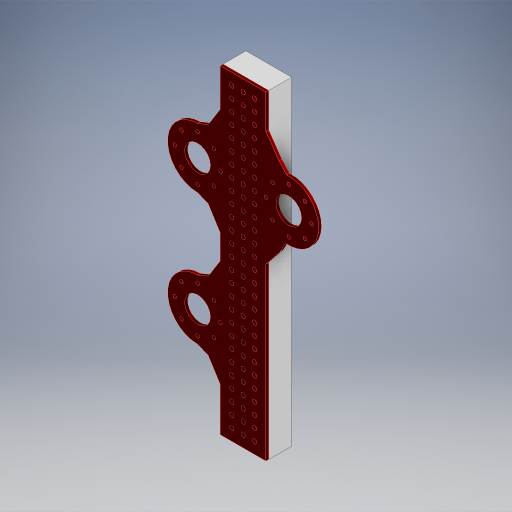
# Autodesk Inventor part: 2024-210-008-Shooter-Gusset-Plate
Saved by Autodesk Inventor 2024.2 (Build 282272000, 272)
## iProperties
Created: 2024-02-16
Part Number: 2024-210-008-Shooter-Gusset-Plate
Material: Generic
Document SubType Name: Modeling
Designer: rohan
Density: 1 g/cm^3
Appearance: Default
Author: rohan
Autodesk Inventor part; units mm, degrees
ref_plane "YZ Plane" through (0, 0, 0) normal (1, 0, 0) x (0, 1, 0)
ref_plane "XZ Plane" through (0, 0, 0) normal (0, 1, 0) x (-1, 0, 0)
ref_plane "XY Plane" through (0, 0, 0) normal (0, 0, 1) x (1, 0, 0)
sketch "Sketch1" plane through (0, 0, 0) normal (0, 1, 0) x (-1, 0, 0)
  line L0 (25.4, 12.7) -> (-25.4, 12.7)
  line L1 (-25.4, 12.7) -> (-25.4, -12.7)
  line L2 (-25.4, -12.7) -> (25.4, -12.7)
  line L3 (25.4, -12.7) -> (25.4, 12.7)
  line L4 (25.4, 12.7) -> (-25.4, -12.7) construction
  line L5 (-25.4, 12.7) -> (25.4, -12.7) construction
  point P0 (0, 0)
  dimension "d0" = 50.8
  dimension "d1" = 25.4
  constraints: 12 end point, 2 midpoint, 2 parallel, 1 horizontal, 1 perpendicular
  measures "d0" distance of L2.end L1.end
  measures "d1" distance of L1.end L0.end
extrude "Extrusion1" add sketch "Sketch1" along normal blind 355.6
sketch "Sketch2" plane through (-25.4, 0, 12.7) normal (0, 0, 1) x (1, 0, 0)
  circle A0 centre (12.7, 12.7) radius 2.4892
  line L0 (0, 0) -> (0, 355.6) projected
  line L1 (0, 0) -> (50.8, 0) projected
  circle A1 centre (25.4, 12.7) radius 2.4892
  circle A2 centre (38.1, 12.7) radius 2.4892
  circle A3 centre (12.7, 25.4) radius 2.4892
  circle A4 centre (25.4, 25.4) radius 2.4892
  circle A5 centre (38.1, 25.4) radius 2.4892
  circle A6 centre (12.7, 38.1) radius 2.4892
  circle A7 centre (25.4, 38.1) radius 2.4892
  circle A8 centre (38.1, 38.1) radius 2.4892
  circle A9 centre (12.7, 50.8) radius 2.4892
  circle A10 centre (25.4, 50.8) radius 2.4892
  circle A11 centre (38.1, 50.8) radius 2.4892
  circle A12 centre (12.7, 63.5) radius 2.4892
  circle A13 centre (25.4, 63.5) radius 2.4892
  circle A14 centre (38.1, 63.5) radius 2.4892
  circle A15 centre (12.7, 76.2) radius 2.4892
  circle A16 centre (25.4, 76.2) radius 2.4892
  circle A17 centre (38.1, 76.2) radius 2.4892
  circle A18 centre (12.7, 88.9) radius 2.4892
  circle A19 centre (25.4, 88.9) radius 2.4892
  circle A20 centre (38.1, 88.9) radius 2.4892
  circle A21 centre (12.7, 101.6) radius 2.4892
  circle A22 centre (25.4, 101.6) radius 2.4892
  circle A23 centre (38.1, 101.6) radius 2.4892
  circle A24 centre (12.7, 114.3) radius 2.4892
  circle A25 centre (25.4, 114.3) radius 2.4892
  circle A26 centre (38.1, 114.3) radius 2.4892
  circle A27 centre (12.7, 127) radius 2.4892
  circle A28 centre (25.4, 127) radius 2.4892
  circle A29 centre (38.1, 127) radius 2.4892
  circle A30 centre (12.7, 139.7) radius 2.4892
  circle A31 centre (25.4, 139.7) radius 2.4892
  circle A32 centre (38.1, 139.7) radius 2.4892
  circle A33 centre (12.7, 152.4) radius 2.4892
  circle A34 centre (25.4, 152.4) radius 2.4892
  circle A35 centre (38.1, 152.4) radius 2.4892
  circle A36 centre (12.7, 165.1) radius 2.4892
  circle A37 centre (25.4, 165.1) radius 2.4892
  circle A38 centre (38.1, 165.1) radius 2.4892
  circle A39 centre (12.7, 177.8) radius 2.4892
  circle A40 centre (25.4, 177.8) radius 2.4892
  circle A41 centre (38.1, 177.8) radius 2.4892
  circle A42 centre (12.7, 190.5) radius 2.4892
  circle A43 centre (25.4, 190.5) radius 2.4892
  circle A44 centre (38.1, 190.5) radius 2.4892
  circle A45 centre (12.7, 203.2) radius 2.4892
  circle A46 centre (25.4, 203.2) radius 2.4892
  circle A47 centre (38.1, 203.2) radius 2.4892
  circle A48 centre (12.7, 215.9) radius 2.4892
  circle A49 centre (25.4, 215.9) radius 2.4892
  circle A50 centre (38.1, 215.9) radius 2.4892
  circle A51 centre (12.7, 228.6) radius 2.4892
  circle A52 centre (25.4, 228.6) radius 2.4892
  circle A53 centre (38.1, 228.6) radius 2.4892
  circle A54 centre (12.7, 241.3) radius 2.4892
  circle A55 centre (25.4, 241.3) radius 2.4892
  circle A56 centre (38.1, 241.3) radius 2.4892
  circle A57 centre (12.7, 254) radius 2.4892
  circle A58 centre (25.4, 254) radius 2.4892
  circle A59 centre (38.1, 254) radius 2.4892
  circle A60 centre (12.7, 266.7) radius 2.4892
  circle A61 centre (25.4, 266.7) radius 2.4892
  circle A62 centre (38.1, 266.7) radius 2.4892
  circle A63 centre (12.7, 279.4) radius 2.4892
  circle A64 centre (25.4, 279.4) radius 2.4892
  circle A65 centre (38.1, 279.4) radius 2.4892
  circle A66 centre (12.7, 292.1) radius 2.4892
  circle A67 centre (25.4, 292.1) radius 2.4892
  circle A68 centre (38.1, 292.1) radius 2.4892
  circle A69 centre (12.7, 304.8) radius 2.4892
  circle A70 centre (25.4, 304.8) radius 2.4892
  circle A71 centre (38.1, 304.8) radius 2.4892
  circle A72 centre (12.7, 317.5) radius 2.4892
  circle A73 centre (25.4, 317.5) radius 2.4892
  circle A74 centre (38.1, 317.5) radius 2.4892
  circle A75 centre (12.7, 330.2) radius 2.4892
  circle A76 centre (25.4, 330.2) radius 2.4892
  circle A77 centre (38.1, 330.2) radius 2.4892
  circle A78 centre (12.7, 342.9) radius 2.4892
  circle A79 centre (25.4, 342.9) radius 2.4892
  circle A80 centre (38.1, 342.9) radius 2.4892
  point P0 (25.4, 0)
  dimension "d4" = 4.9784
  dimension "d5" = 12.7
  dimension "d6" = 12.7
  dimension "d9" = 12.7
  dimension "d12" = 12.7
  constraints: 81 centre point, 1 horizontal, 1 vertical, 160 other
  measures "d4" diameter of A0
  measures "d5" distance from line of A0.centre L1
  measures "d6" distance from line of L0 A0.centre
  measures "d9" distance of A0.centre A1.centre
  measures "d12" distance of A0.centre A3.centre
extrude "Extrusion2" cut sketch "Sketch2" against normal blind 355.6
sketch "Sketch3" plane through (-25.4, 0, 12.7) normal (0, 0, 1) x (1, 0, 0)
  circle A0 centre (38.1, 342.9) radius 2.4892 projected
  circle A1 centre (12.7, 317.5) radius 2.4892 projected
  circle A2 centre (12.7, 292.1) radius 2.4892 projected
  circle A3 centre (38.1, 266.7) radius 2.4892 projected
  circle A4 centre (25.4, 304.8) radius 2.4892 projected
  circle A5 centre (12.7, 241.3) radius 2.4892 projected
  circle A6 centre (38.1, 215.9) radius 2.4892 projected
  circle A7 centre (38.1, 254) radius 2.4892 projected
  circle A8 centre (25.4, 203.2) radius 2.4892 projected
  circle A9 centre (38.1, 177.8) radius 2.4892 projected
  circle A10 centre (38.1, 165.1) radius 2.4892 projected
  circle A11 centre (12.7, 165.1) radius 2.4892 projected
  circle A12 centre (25.4, 127) radius 2.4892 projected
  circle A13 centre (38.1, 114.3) radius 2.4892 projected
  circle A14 centre (12.7, 88.9) radius 2.4892 projected
  circle A15 centre (25.4, 101.6) radius 2.4892 projected
  circle A16 centre (38.1, 63.5) radius 2.4892 projected
  circle A17 centre (12.7, 50.8) radius 2.4892 projected
  circle A18 centre (38.1, 12.7) radius 2.4892 projected
  circle A19 centre (12.7, 38.1) radius 2.4892 projected
  circle A20 centre (25.4, 38.1) radius 2.4892 projected
  circle A21 centre (25.4, 12.7) radius 2.4892 projected
  circle A22 centre (12.7, 63.5) radius 2.4892 projected
  circle A23 centre (38.1, 50.8) radius 2.4892 projected
  circle A24 centre (38.1, 101.6) radius 2.4892 projected
  circle A25 centre (12.7, 76.2) radius 2.4892 projected
  circle A26 centre (25.4, 114.3) radius 2.4892 projected
  circle A27 centre (25.4, 139.7) radius 2.4892 projected
  circle A28 centre (12.7, 152.4) radius 2.4892 projected
  circle A29 centre (38.1, 152.4) radius 2.4892 projected
  circle A30 centre (25.4, 177.8) radius 2.4892 projected
  circle A31 centre (38.1, 203.2) radius 2.4892 projected
  circle A32 centre (25.4, 254) radius 2.4892 projected
  circle A33 centre (38.1, 228.6) radius 2.4892 projected
  circle A34 centre (12.7, 228.6) radius 2.4892 projected
  circle A35 centre (38.1, 292.1) radius 2.4892 projected
  circle A36 centre (25.4, 279.4) radius 2.4892 projected
  circle A37 centre (12.7, 279.4) radius 2.4892 projected
  circle A38 centre (25.4, 317.5) radius 2.4892 projected
  circle A39 centre (12.7, 330.2) radius 2.4892 projected
  circle A40 centre (25.4, 342.9) radius 2.4892 projected
  circle A41 centre (38.1, 330.2) radius 2.4892 projected
  circle A42 centre (12.7, 304.8) radius 2.4892 projected
  circle A43 centre (25.4, 266.7) radius 2.4892 projected
  circle A44 centre (25.4, 292.1) radius 2.4892 projected
  circle A45 centre (12.7, 254) radius 2.4892 projected
  circle A46 centre (25.4, 215.9) radius 2.4892 projected
  circle A47 centre (38.1, 241.3) radius 2.4892 projected
  circle A48 centre (12.7, 203.2) radius 2.4892 projected
  circle A49 centre (25.4, 190.5) radius 2.4892 projected
  circle A50 centre (38.1, 190.5) radius 2.4892 projected
  circle A51 centre (25.4, 152.4) radius 2.4892 projected
  circle A52 centre (12.7, 127) radius 2.4892 projected
  circle A53 centre (38.1, 127) radius 2.4892 projected
  circle A54 centre (12.7, 101.6) radius 2.4892 projected
  circle A55 centre (25.4, 88.9) radius 2.4892 projected
  circle A56 centre (38.1, 76.2) radius 2.4892 projected
  circle A57 centre (25.4, 63.5) radius 2.4892 projected
  circle A58 centre (38.1, 25.4) radius 2.4892 projected
  circle A59 centre (12.7, 25.4) radius 2.4892 projected
  circle A60 centre (25.4, 25.4) radius 2.4892 projected
  circle A61 centre (12.7, 12.7) radius 2.4892 projected
  circle A62 centre (38.1, 38.1) radius 2.4892 projected
  circle A63 centre (25.4, 50.8) radius 2.4892 projected
  circle A64 centre (38.1, 88.9) radius 2.4892 projected
  circle A65 centre (25.4, 76.2) radius 2.4892 projected
  circle A66 centre (12.7, 114.3) radius 2.4892 projected
  circle A67 centre (38.1, 139.7) radius 2.4892 projected
  circle A68 centre (12.7, 139.7) radius 2.4892 projected
  circle A69 centre (25.4, 165.1) radius 2.4892 projected
  circle A70 centre (12.7, 177.8) radius 2.4892 projected
  circle A71 centre (12.7, 190.5) radius 2.4892 projected
  circle A72 centre (25.4, 228.6) radius 2.4892 projected
  circle A73 centre (25.4, 241.3) radius 2.4892 projected
  circle A74 centre (12.7, 215.9) radius 2.4892 projected
  circle A75 centre (38.1, 304.8) radius 2.4892 projected
  circle A76 centre (38.1, 279.4) radius 2.4892 projected
  circle A77 centre (12.7, 266.7) radius 2.4892 projected
  circle A78 centre (38.1, 317.5) radius 2.4892 projected
  circle A79 centre (25.4, 330.2) radius 2.4892 projected
  circle A80 centre (12.7, 342.9) radius 2.4892 projected
  line L0 (0, 0) -> (50.8, 0) projected
  line L1 (50.8, 0) -> (50.8, 355.6) projected
  line L2 (0, 355.6) -> (50.8, 355.6) projected
  line L3 (0, 0) -> (0, 355.6) projected
  circle A81 centre (76.1238, 254) radius 14.2748
  circle A82 centre (-25.2476, 254) radius 14.2748
  circle A83 centre (-25.2476, 107.95) radius 14.2748
  circle A84 centre (76.1238, 279.4) radius 2.0193
  circle A85 centre (76.1238, 228.6) radius 2.0193
  circle A86 centre (-25.2476, 279.4) radius 2.0193
  circle A87 centre (-50.6476, 254) radius 2.0193
  circle A88 centre (-25.2476, 228.6) radius 2.0193
  circle A89 centre (0.1524, 254) radius 2.0193
  circle A90 centre (-25.2476, 133.35) radius 2.0193
  circle A91 centre (-50.6476, 107.95) radius 2.0193
  circle A92 centre (-25.2476, 82.55) radius 2.0193
  circle A93 centre (0.1524, 107.95) radius 2.0193
  circle A94 centre (-25.2476, 254) radius 33.3248
  circle A95 centre (76.1238, 254) radius 33.3248
  circle A96 centre (-25.2476, 107.95) radius 33.3248
  line L4 (73.8666, 287.2483) -> (65.2991, 296.6231)
  line L5 (65.2991, 296.6231) -> (50.8, 317.4782)
  line L6 (50.8, 0) -> (50.8, 355.6) projected
  line L7 (72.7187, 220.8496) -> (66.6451, 209.6961)
  line L8 (66.6451, 209.6961) -> (50.8, 189.8443)
  line L9 (-25.2476, 287.3248) -> (-13.4795, 292.1)
  line L10 (-13.4795, 292.1) -> (0, 313.6282)
  line L11 (0, 0) -> (0, 355.6) projected
  line L12 (-25.2476, 220.6752) -> (-13.4795, 215.9)
  line L13 (-13.4795, 215.9) -> (0, 194.3718)
  line L14 (-25.2476, 141.2748) -> (-13.4795, 146.0434)
  line L15 (-13.4795, 146.0434) -> (0, 167.5715)
  line L16 (-25.2476, 74.6252) -> (-13.4795, 69.85)
  line L17 (-13.4795, 69.85) -> (0, 48.3218)
  circle A97 centre (-7.2871, 89.9895) radius 2.0193
  circle A98 centre (0.1524, 107.95) radius 2.0193
  circle A99 centre (-7.2871, 125.9105) radius 2.0193
  circle A100 centre (-25.2476, 133.35) radius 2.0193
  circle A101 centre (-43.2081, 125.9105) radius 2.0193
  circle A102 centre (-50.6476, 107.95) radius 2.0193
  circle A103 centre (-43.2081, 89.9895) radius 2.0193
  circle A104 centre (-7.2871, 236.0395) radius 2.0193
  circle A105 centre (0.1524, 254) radius 2.0193
  circle A106 centre (-7.2871, 271.9605) radius 2.0193
  circle A107 centre (-25.2476, 279.4) radius 2.0193
  circle A108 centre (-43.2081, 271.9605) radius 2.0193
  circle A109 centre (-50.6476, 254) radius 2.0193
  circle A110 centre (-43.2081, 236.0395) radius 2.0193
  circle A111 centre (94.0843, 236.0395) radius 2.0193
  circle A112 centre (101.5238, 254) radius 2.0193
  circle A113 centre (94.0843, 271.9605) radius 2.0193
  circle A114 centre (76.1238, 279.4) radius 2.0193
  circle A115 centre (58.1633, 271.9605) radius 2.0193
  circle A116 centre (50.7238, 254) radius 2.0193
  circle A117 centre (58.1633, 236.0395) radius 2.0193
  point P0 (25.4, 0)
  point P1 (0, 232.2491)
  point P2 (0, 129.7009)
  point P3 (0, 86.1991)
  point P4 (50.8, 232.3379)
  point P5 (50.8, 275.6621)
  point P6 (0, 275.7509)
  point P7 (50.8, 317.4782)
  dimension "d17" = 28.5496
  dimension "d18" = 101.6
  dimension "d19" = 28.5496
  dimension "d20" = 101.6
  dimension "d21" = 101.3714
  dimension "d22" = 25.2476
  dimension "d23" = 28.5496
  dimension "d24" = 146.05
  dimension "d25" = 4.0386
  dimension "d26" = 4.0386
  dimension "d27" = 50.8
  dimension "d28" = 25.4
  dimension "d33" = 25.4
  dimension "d36" = 360
  dimension "d38" = 4.0386
  dimension "d39" = 25.4
  dimension "d42" = 360
  dimension "d44" = 19.05
  dimension "d45" = 19.05
  dimension "d46" = 19.05
  dimension "d47" = 12.7
  dimension "d48" = 25.4
  dimension "d49" = 12.7
  dimension "d50" = 25.4
  dimension "d51" = 12.7
  dimension "d52" = 25.4
  dimension "d53" = 12.7
  dimension "d54" = 25.4
  dimension "d56" = 25.4
  dimension "d57" = 12.7
  dimension "d58" = 25.4
  dimension "d63" = 360
  dimension "d67" = 360
  dimension "d75" = 360
  constraints: 37 centre point, 24 end point, 6 point on circle, 6 point on line, 69 other
  measures "d17" diameter of A81
  measures "d18" distance from line of A81.centre L2
  measures "d19" diameter of A82
  measures "d20" distance from line of L2 A82.centre
  measures "d21" distance of A81.centre A82.centre
  measures "d22" distance from line of L3 A82.centre
  measures "d23" diameter of A83
  measures "d24" distance of A83.centre A82.centre
  measures "d25" diameter of A84
  measures "d26" diameter of A85
  measures "d27" distance of A84.centre A85.centre
  measures "d28" distance of A81.centre A84.centre
  measures "d33" distance of A82.centre A86.centre
  measures "d38" diameter of A90
  measures "d39" distance of A83.centre A90.centre
  measures "d44" radial gap between concentric circles of A82 A94
  measures "d45" radial gap between concentric circles of A81 A95
  measures "d46" radial gap between concentric circles of A83 A96
  measures "d47" distance of L4.start L4.end
  measures "d48" distance of L4.end L5.end
  measures "d49" distance of L7.start L7.end
  measures "d50" distance of L7.end L8.end
  measures "d51" distance of L9.start L9.end
  measures "d52" distance of L9.end L10.end
  measures "d53" distance of L12.start L12.end
  measures "d54" distance of L12.end L13.end
  measures "d56" distance of L14.end L15.end
  measures "d57" distance of L16.start L16.end
  measures "d58" distance of L16.end L17.end
extrude "Extrusion3" add sketch "Sketch3" along normal blind 3.175 separate body contours L3 A96 A94 L2 L1 A95 L0 | L17 L16 A96 L3 | L1 A95 L7 L8 | A96 L3 A93 | L3 A93 A96 | A95 L1 A116 | L1 A116 A95 | L1 L5 L4 A95 | L14 L15 L3 A96 | L13 L12 A94 L3 | A94 L3 A89 | L3 A89 A94 | L3 A94 L9 L10
body "Solid1"
